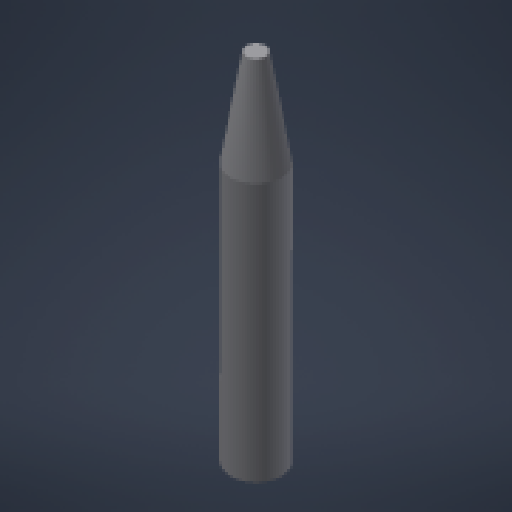
# Autodesk Inventor part: Stand
Saved by Autodesk Inventor 2026.1 (Build 301233000, 233)
## iProperties
Manager: MANUTENÇÃO GUIFÕES - CP
Company: CP
Created: 2025-09-03
Part Number: Stand
Project: 0.00 0000/00
Checked By: PMFIGUEIREDO
Engr Approved By: JSSILVA
Material: Generic
Description: NOME DA PEÇA
Document SubType Name: Modeling
Designer: TPMIRANDA
Engineer: ISO 2768 - m K
Authority: Nº DESENHO PELO QUAL FOI SUBSITUIDO
Stock Number: 00000-000
Density: 1 g/cm^3
Appearance: Default
Title: UME 3400
Subject: CAIXA, INTERIOR, SUPORTE,
Author: TPMIRANDA
Keywords: Caixa de comentários. Substituir texto, ou eliminar.
Comments: UQE2300 UQE2400 UTE2240 UDD9630 CARRUAGENS SIMAFE CARRUAGENS CAF CARRUAGENS ARCO
Revision Number: Nº DESENHO QUE SUBSTITUI
Autodesk Inventor part; units mm, degrees
ref_plane "YZ Plane" through (0, 0, 0) normal (1, 0, 0) x (0, 1, 0)
ref_plane "XZ Plane" through (0, 0, 0) normal (0, 1, 0) x (-1, 0, 0)
sketch "Sketch1" plane through (0, 0, 0) normal (0, 0, 1) x (1, 0, 0)
  circle A0 centre (0, 0) radius 0.4
  dimension "d0" = 0.8
  constraints: 1 centre point, 1 coincident
  measures "d0" diameter of A0
extrude "Extrusion1" add sketch "Sketch1" along normal blind 4
sketch "Sketch2" plane through (0, 0, 4) normal (0, 0, 1) x (1, 0, 0)
  circle A0 centre (0, 0) radius 0.4 projected
ref_plane "Work Plane1" through (0, 0, 5.5) normal (0, 0, 1) x (1, 0, 0)
sketch "Sketch3" plane through (0, 0, 5.5) normal (0, 0, 1) x (1, 0, 0)
  circle A0 centre (0, 0) radius 0.15
  dimension "d4" = 0.3
  constraints: 1 centre point, 1 coincident
  measures "d4" diameter of A0
loft "Loft1" add profiles "Sketch2", "Sketch3"
body "Solid1"
